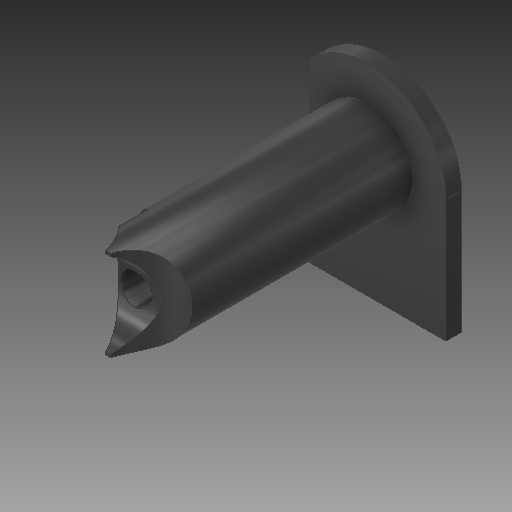
# Autodesk Inventor part: guide tube
Saved by Autodesk Inventor 2018 (Build 220112000, 112)
## iProperties
Created: 2016-06-27
Part Number: guide tube
Material: Generic
Document SubType Name: Modeling
Designer: Ben
Density: 1 g/cm^3
Appearance: Default
Author: Ben
Autodesk Inventor part; units mm, degrees
ref_plane "YZ Plane" through (0, 0, 0) normal (1, 0, 0) x (0, 1, 0)
ref_plane "XZ Plane" through (0, 0, 0) normal (0, 1, 0) x (-1, 0, 0)
ref_plane "XY Plane" through (0, 0, 0) normal (0, 0, 1) x (1, 0, 0)
sketch "Sketch1" plane through (0, 0, 0) normal (0, 0, 1) x (1, 0, 0)
  circle A0 centre (0, 0) radius 3.625
  dimension "d0" = 7.25
  constraints: 1 centre point, 1 coincident
  measures "d0" diameter of A0
extrude "Extrusion1" add sketch "Sketch1" along normal blind 22
sketch "Sketch2" plane through (0, 0, 0) normal (0, 0, -1) x (-1, 0, 0)
  arc A0 (4.6, 4.3046) -> (-6.3, 0) centre (0, 0) ccw
  line L0 (4.6, 4.3046) -> (4.6, -9.8)
  line L1 (-6.3, 0) -> (-6.3, -9.8)
  line L2 (-6.3, -9.8) -> (4.6, -9.8)
  dimension "d3" = 6.3
  dimension "d4" = 4.6
  dimension "d5" = 9.8
  constraints: 6 end point, 2 point on circle, 2 vertical, 1 centre point, 1 coincident, 1 perpendicular, 1 tangent
  measures "d3" radius of A0
  measures "d4" distance from line of point (0, 0) L0
  measures "d5" distance from line of point (0, 0) L2
extrude "Extrusion2" add sketch "Sketch2" against normal blind 1.25
sketch "Sketch3" plane through (0, 0, 0) normal (0, 0, -1) x (-1, 0, 0)
  circle A0 centre (0, 0) radius 2.2
  dimension "d8" = 4.4
  constraints: 1 centre point, 1 coincident
  measures "d8" diameter of A0
extrude "Extrusion3" cut sketch "Sketch3" against normal blind 16
sketch "Sketch4" plane through (0, 0, 22) normal (0, 0, 1) x (1, 0, 0)
  circle A0 centre (0, 0) radius 2.2 projected
  circle A1 centre (0, 0) radius 1.25
  dimension "d11" = 2.5
  constraints: 1 centre point, 1 coincident
  measures "d11" diameter of A1
extrude "Extrusion4" cut sketch "Sketch4" against normal up to next contours A1
chamfer "Chamfer1" distance 1.4 angle 45 1 edges at (2.2, 0, 0)
sketch "Sketch5" plane through (0, 0, 0) normal (0, 1, 0) x (-1, 0, 0)
  line L0 (3.625, 1.25) -> (3.625, 22) projected
  line L1 (-3.625, 1.25) -> (-3.625, 22) projected
  line L2 (3.625, 22) -> (-3.625, 22) projected
  line L3 (3.625, 17) -> (1.8, 17)
  line L4 (1.8, 17) -> (1.8, 22)
  line L5 (1.8, 22) -> (3.625, 22)
  line L6 (3.625, 22) -> (3.625, 17)
  line L7 (-3.6, 0) -> (3.6, 0) projected
  line L8 (1.8, 17) -> (3.625, 15.9463)
  line L9 (3.625, 1.25) -> (3.625, 22) projected
  line L10 (1.8, 17) -> (3.9073, 17) construction
  line L11 (3.625, 15.9463) -> (3.625, 17)
  point P0 (0, 0)
  dimension "d17" = 5.425
  dimension "d18" = 17
  dimension "d21" = 30
  constraints: 14 end point, 3 point on line, 2 horizontal, 2 parallel, 1 collinear, 1 equal length, 1 perpendicular
  measures "d17" distance between parallel lines of L1 L4
  measures "d18" distance between parallel lines of L7 L3
  measures "d21" angle of L8 L10
extrude "Extrusion5" cut sketch "Sketch5" along normal through all both and the other way through all
sketch "Sketch6" plane through (0, 0, 0) normal (0, 1, 0) x (-1, 0, 0)
  line L0 (1.8, 22) -> (-3.625, 22) projected
  line L1 (-1.25, 22) -> (1.25, 22) projected
  line L2 (0, 22) -> (0, 19.2621) construction
  circle A0 centre (-4.6, 23.4) radius 4.6
  circle A1 centre (5.4, 23.4) radius 5.4
  line L3 (12.1762, 23.4) -> (-11.9471, 23.4)
  point P0 (0, 0)
  dimension "d22" = 4.6
  dimension "d23" = 5.4
  dimension "d24" = 1.4
  constraints: 4 end point, 2 centre point, 2 point on line, 2 tangent, 1 horizontal, 1 midpoint, 1 vertical
  measures "d22" distance from line of L2 A0.centre
  measures "d23" distance from line of L2 A1.centre
  measures "d24" distance between parallel lines of L0 L3
extrude "Extrusion6" cut sketch "Sketch6" along normal through all both and the other way through all contours A1 L3 | A0 L3 | L3 A0 | A1 L3
sketch "Sketch7" plane through (0, 0, 0) normal (1, 0, 0) x (0, 1, 0)
  line L0 (-3.1465, 19.3751) -> (3.1465, 19.3751) projected
  line L1 (1.2308, 22) -> (3.6184, 22) projected
  line L2 (3.6184, 22) -> (3.6184, 24.6476)
  line L3 (0, 19.6751) -> (0, 24.6476) construction
  circle A0 centre (0, 23.2935) radius 3.6184
  point P0 (0, 0)
  point P1 (0, 19.3751)
  dimension "d29" = 0.3
  constraints: 4 end point, 3 vertical, 2 point on line, 1 midpoint, 1 vertical alignment, 2 other
  measures "d29" distance from line of L0 L3.start
extrude "Extrusion7" cut sketch "Sketch7" along normal through all both and the other way through all contours A0
body "Solid1"
